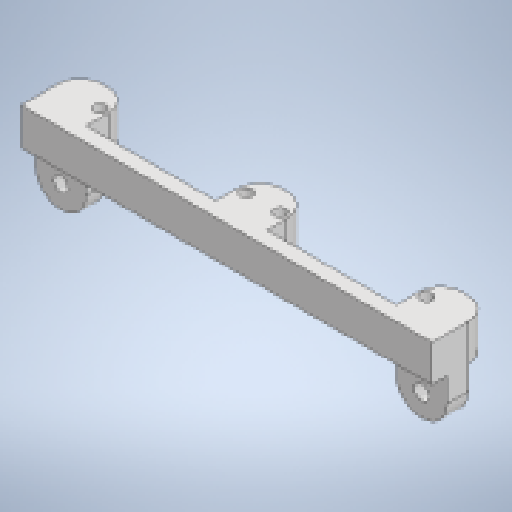
# Autodesk Inventor part: mocowanie_serw
Saved by Autodesk Inventor 2023 (Build 270158000, 158)
## iProperties
Created: 2023-04-06
Part Number: mocowanie_serw
Material: Ogólny
Document SubType Name: Modeling
Designer: Kamil
Density: 1 g/cm^3
Appearance: Domyślna
Author: Kamil
Autodesk Inventor part; units mm, degrees
ref_plane "YZ Plane" through (0, 0, 0) normal (1, 0, 0) x (0, 1, 0)
ref_plane "XZ Plane" through (0, 0, 0) normal (0, 1, 0) x (-1, 0, 0)
ref_plane "XY Plane" through (0, 0, 0) normal (0, 0, 1) x (1, 0, 0)
sketch "Szkic1" plane through (0, 0, 0) normal (0, 0, 1) x (1, 0, 0)
  arc A0 (-14.5572, 8.86) -> (-14.6986, 8.8014) centre (-14.5572, 8.66) ccw projected
  line L0 (-15.5414, 7.9586) -> (-14.6986, 8.8014) projected
  arc A1 (-15.6828, 7.9) -> (-15.5414, 7.9586) centre (-15.6828, 8.1) ccw projected
  line L1 (-16.4, 7.9) -> (-15.6828, 7.9) projected
  line L2 (-16.4, 7.9) -> (-16.4, 6.8) projected
  arc A2 (-16.4, 6.8) -> (-16.2, 6.6) centre (-16.2, 6.8) ccw projected
  line L3 (-16.2, 6.6) -> (-11.8, 6.6) projected
  line L4 (-11.8, 6.6) -> (-11.8, -11.6) projected
  line L5 (-11.8, -11.6) -> (11.8, -11.6) projected
  line L6 (11.8, -11.6) -> (11.8, 6.6) projected
  line L7 (11.8, 6.6) -> (16.2, 6.6) projected
  arc A3 (16.2, 6.6) -> (16.4, 6.8) centre (16.2, 6.8) ccw projected
  line L8 (16.4, 6.8) -> (16.4, 7.9) projected
  line L9 (16.4, 7.9) -> (15.7657, 7.9) projected
  arc A4 (15.4828, 8.0172) -> (15.7657, 7.9) centre (15.7657, 8.3) ccw projected
  line L10 (15.4828, 8.0172) -> (14.6986, 8.8014) projected
  arc A5 (14.6986, 8.8014) -> (14.5572, 8.86) centre (14.5572, 8.66) ccw projected
  line L11 (11.8, 8.86) -> (14.5572, 8.86) projected
  line L12 (11.8, 8.86) -> (11.8, 11.6) projected
  line L13 (11.8, 11.6) -> (8.3794, 11.6) projected
  line L14 (8.3794, 11.6) -> (8.3794, 16) projected
  line L15 (8.3794, 16) -> (4.0206, 16) projected
  line L16 (4.0206, 11.6) -> (4.0206, 16) projected
  line L17 (4.0206, 11.6) -> (-11.8, 11.6) projected
  line L18 (-11.8, 11.6) -> (-11.8, 8.86) projected
  line L19 (-11.8, 8.86) -> (-14.5572, 8.86) projected
  arc A6 (51.4986, 8.8014) -> (51.3572, 8.86) centre (51.3572, 8.66) ccw projected
  line L20 (48.6, 8.86) -> (51.3572, 8.86) projected
  line L21 (48.6, 11.6) -> (48.6, 8.86) projected
  line L22 (32.7794, 11.6) -> (48.6, 11.6) projected
  line L23 (32.7794, 11.6) -> (32.7794, 16) projected
  line L24 (28.4206, 16) -> (32.7794, 16) projected
  line L25 (28.4206, 11.6) -> (28.4206, 16) projected
  line L26 (25, 11.6) -> (28.4206, 11.6) projected
  line L27 (25, 8.86) -> (25, 11.6) projected
  line L28 (25, 8.86) -> (22.2428, 8.86) projected
  arc A7 (22.2428, 8.86) -> (22.1014, 8.8014) centre (22.2428, 8.66) ccw projected
  line L29 (21.3172, 8.0172) -> (22.1014, 8.8014) projected
  arc A8 (21.0343, 7.9) -> (21.3172, 8.0172) centre (21.0343, 8.3) ccw projected
  line L30 (20.4, 7.9) -> (21.0343, 7.9) projected
  line L31 (20.4, 6.8) -> (20.4, 7.9) projected
  arc A9 (20.4, 6.8) -> (20.6, 6.6) centre (20.6, 6.8) ccw projected
  line L32 (25, 6.6) -> (20.6, 6.6) projected
  line L33 (25, -11.6) -> (25, 6.6) projected
  line L34 (48.6, -11.6) -> (25, -11.6) projected
  line L35 (48.6, 6.6) -> (48.6, -11.6) projected
  line L36 (53, 6.6) -> (48.6, 6.6) projected
  arc A10 (53, 6.6) -> (53.2, 6.8) centre (53, 6.8) ccw projected
  line L37 (53.2, 7.9) -> (53.2, 6.8) projected
  line L38 (53.2, 7.9) -> (52.4828, 7.9) projected
  arc A11 (52.3414, 7.9586) -> (52.4828, 7.9) centre (52.4828, 8.1) ccw projected
  line L39 (52.3414, 7.9586) -> (51.4986, 8.8014) projected
  line L40 (-23.6, -41.4743) -> (-23.6, 10.2735) projected
  line L41 (60.4, -41.4743) -> (60.4, 10.2735) projected
  line L42 (-12.3, 19.2958) -> (-12.3, -9.7042) projected
  line L43 (-12.1464, 6.4) -> (-16.2, 6.4) projected
  line L44 (11.8, 6.6) -> (16.2, 6.6) projected
  line L45 (16.2, 6.4) -> (12.1464, 6.4) projected
  line L46 (12.2, 6.4) -> (12.2, -11.6) projected
  line L47 (24.6, 6.4) -> (24.6, -11.6) projected
  line L48 (20.6, 6.4) -> (24.6536, 6.4) projected
  line L49 (12.2, 6.4) -> (24.6, 6.4)
  line L50 (24.6, 6.4) -> (24.6, -11.6)
  line L51 (24.6, -11.6) -> (12.2, -11.6)
  line L52 (12.2, -11.6) -> (12.2, 6.4)
  line L53 (-12.3, 6.4) -> (-23.6, 6.4)
  line L54 (-23.6, 6.4) -> (-23.6, -11.6)
  line L55 (-23.6, -11.6) -> (-12.3, -11.6)
  line L56 (-12.3, -11.6) -> (-12.3, 6.4)
  line L57 (18.4, 10.2735) -> (18.4, 28.3356)
  line L58 (49.1, 6.4) -> (60.4, 6.4)
  line L59 (60.4, 6.4) -> (60.4, -11.6)
  line L60 (60.4, -11.6) -> (49.1, -11.6)
  line L61 (49.1, -11.6) -> (49.1, 6.4)
  line L62 (59.4, 5.4) -> (50.1, 5.4)
  line L63 (50.1, 5.4) -> (50.1, -10.6)
  line L64 (50.1, -10.6) -> (59.4, -10.6)
  line L65 (59.4, -10.6) -> (59.4, 5.4)
  line L66 (13.2, -10.6) -> (23.6, -10.6)
  line L67 (23.6, -10.6) -> (23.6, 5.4)
  line L68 (23.6, 5.4) -> (13.2, 5.4)
  line L69 (13.2, 5.4) -> (13.2, -10.6)
  line L70 (-13.3, -10.6) -> (-22.6, -10.6)
  line L71 (-22.6, -10.6) -> (-22.6, 5.4)
  line L72 (-22.6, 5.4) -> (-13.3, 5.4)
  line L73 (-13.3, 5.4) -> (-13.3, -10.6)
  line L74 (59.4, -10.6) -> (62.4536, -10.6)
  line L75 (59.4, 5.4) -> (62.0484, 5.4)
  line L76 (-22.6, -10.6) -> (-26.8003, -10.6)
  line L77 (-22.6, 5.4) -> (-29.2872, 5.4)
  point P0 (0, 0)
  point P1 (60.4, -10.6)
  point P2 (60.4, 5.4)
  point P3 (-23.6, 5.4)
  point P4 (-23.6, -10.6)
  dimension "d0" = 1
  dimension "d1" = 1
  dimension "d2" = 1
  constraints: 58 end point, 8 parallel, 5 horizontal, 5 perpendicular, 4 symmetric about line, 3 point on line, 1 vertical, 9 other
  measures "d0" distance between parallel lines of L58 L62
  measures "d1" distance between parallel lines of L51 L66
  measures "d2" distance between parallel lines of L55 L70
ref_plane "Płaszczyzna konstrukcyjna1" through (20.4, -11.6, -9) normal (0, 0, -1) x (0, 1, 0)
extrude "Wyciągnięcie proste1" add sketch "Szkic1" against normal up to surface (9 mm away) contours L40 L77 L71 L76 | L71 L72 L73 L70 | L74 L65 L75 L41 | L64 L63 L62 L65 | L69 L68 L67 L66
sketch "Szkic2" plane through (0, 0, 0) normal (0, 0, 1) x (1, 0, 0)
  line L0 (-23.6, 5.4) -> (-23.6, -10.6) projected
  line L1 (-23.6, -10.6) -> (-13.3, -10.6) projected
  line L2 (-13.3, -10.6) -> (-13.3, 5.4) projected
  line L3 (-13.3, 5.4) -> (-23.6, 5.4) projected
  line L4 (50.1, 5.4) -> (50.1, -10.6) projected
  line L5 (50.1, -10.6) -> (60.4, -10.6) projected
  line L6 (60.4, -10.6) -> (60.4, 5.4) projected
  line L7 (60.4, 5.4) -> (50.1, 5.4) projected
  line L8 (23.6, -10.6) -> (23.6, 5.4) projected
  line L9 (23.6, 5.4) -> (13.2, 5.4) projected
  line L10 (13.2, 5.4) -> (13.2, -10.6) projected
  line L11 (13.2, -10.6) -> (23.6, -10.6) projected
  line L12 (-23.6, -10.6) -> (60.4, -10.6)
  line L13 (60.4, -10.6) -> (60.4, 5.4)
  line L14 (60.4, 5.4) -> (-23.6, 5.4)
  line L15 (-23.6, 5.4) -> (-23.6, -10.6)
  point P0 (0, 0)
  constraints: 8 end point, 2 parallel, 1 horizontal, 1 perpendicular
ref_plane "Płaszczyzna konstrukcyjna2" through (60.4, -41.4743, 3) normal (0, 0, 1) x (1, 0, 0)
extrude "Wyciągnięcie proste2" add sketch "Szkic2" along normal up to surface (3 mm away)
sketch "Szkic3" plane through (13.2, -10.6, -9) normal (0, -1, 0) x (1, 0, 0)
  line L0 (36.9, 0) -> (47.2, 0) projected
  line L1 (47.2, 0) -> (47.2, 12) projected
  line L2 (47.2, 12) -> (-36.8, 12) projected
  line L3 (-36.8, 0) -> (-36.8, 12) projected
  line L4 (-36.8, 0) -> (-26.5, 0) projected
  line L5 (-26.5, 9) -> (-26.5, 0) projected
  line L6 (-26.5, 9) -> (0, 9) projected
  line L7 (0, 9) -> (0, 0) projected
  line L8 (0, 0) -> (10.4, 0) projected
  line L9 (10.4, 9) -> (10.4, 0) projected
  line L10 (10.4, 9) -> (36.9, 9) projected
  line L11 (36.9, 9) -> (36.9, 0) projected
  point P0 (-13.2, 9)
extrude "Wyciągnięcie proste3" cut sketch "Szkic3" against normal blind 5
move faces "Przesuń1" translate (0, 1, 0) faces at (28.9667, -5.6, 2)
sketch "Szkic4" plane through (-23.6, -4.6, 3) normal (0, -1, 0) x (1, 0, 0)
  line L0 (74.8605, -3) -> (10.8605, -3) projected
  line L1 (36.8, -12) -> (36.8, -3) projected
  line L2 (47.2, -3) -> (47.2, -12) projected
  line L3 (47.2, -12) -> (36.8, -12) projected
  point P0 (23.6, -3)
ref_plane "Płaszczyzna konstrukcyjna3" through (-11.8, -12, -8.6) normal (0, -1, 0) x (1, 0, 0)
extrude "Wyciągnięcie proste4" add sketch "Szkic4" along normal up to surface (7.4 mm away)
move faces "Przesuń2" translate (0, 2.5, 0) faces at (7.8333, -4.6, 2)
sketch "Szkic5" plane through (13.2, -12, 0) normal (0, 0, 1) x (1, 0, 0)
  line L0 (-36.8, 9.9) -> (47.2, 9.9) projected
  line L1 (0, 9.9) -> (0, 0) projected
  line L2 (0, 0) -> (10.4, 0) projected
  line L3 (10.4, 9.9) -> (10.4, 0) projected
  line L4 (10.4, 0) -> (0, 0) projected
  line L5 (5.2, 0) -> (5.2, 7.1911)
  line L6 (0, 4.95) -> (10.4, 4.95)
  line L7 (10.4, 0) -> (10.4, 17.4) projected
  circle A0 centre (5.2, 4.95) radius 1.5
  point P0 (-13.2, 12)
  dimension "d17" = 3
  constraints: 4 end point, 3 midpoint, 1 centre point, 1 horizontal, 1 point on line, 1 vertical
  measures "d17" diameter of A0
extrude "Wyciągnięcie proste5" cut sketch "Szkic5" against normal through all contours A0 L5 L6 | L6 L5 A0 | A0 L5 L6 | L6 L5 A0
sketch "Szkic6" plane through (-23.6, -2.1, 3) normal (0, -1, 0) x (1, 0, 0)
  line L0 (36.8, -3) -> (47.2, -3) projected
  line L1 (73.7, -3) -> (47.2, -3) projected
  line L2 (73.7, -12) -> (73.7, -3) projected
  line L3 (84, -12) -> (73.7, -12) projected
  line L4 (84, 0) -> (84, -12) projected
  line L5 (0, 0) -> (84, 0) projected
  line L6 (0, -12) -> (0, 0) projected
  line L7 (10.3, -12) -> (0, -12) projected
  line L8 (10.3, -3) -> (10.3, -12) projected
  line L9 (36.8, -3) -> (10.3, -3) projected
  line L10 (0, -3) -> (84, -3)
  line L11 (84, -3) -> (84, -12)
  line L12 (84, -12) -> (0, -12)
  line L13 (0, -12) -> (0, -3)
  line L14 (84, -12) -> (84, 0) projected
  line L15 (0, -3) -> (84, -3)
  line L16 (84, -3) -> (84, -7.5)
  line L17 (84, -7.5) -> (0, -7.5)
  line L18 (0, -7.5) -> (0, -3)
  point P0 (23.6, -3)
  point P1 (73.7, -7.5)
  point P2 (73.7, -3)
  point P3 (0, -7.5)
  point P4 (10.3, -7.5)
  constraints: 16 end point, 4 parallel, 2 horizontal, 2 perpendicular, 2 point on line
extrude "Wyciągnięcie proste6" add sketch "Szkic6" along normal up to surface (9.9 mm away) contours L8 L17 L6 L10 | L10 L4 L17 L2
sketch "Szkic7" plane through (13.2, -12, 0) normal (0, 0, 1) x (1, 0, 0)
  circle A0 centre (5.2, 4.95) radius 1.5 projected
  line L0 (0, 0) -> (10.4, 0) projected
  line L1 (10.4, 9.9) -> (10.4, 0) projected
  line L2 (0, 9.9) -> (10.4, 9.9) projected
  line L3 (0, 9.9) -> (0, 0) projected
  point P0 (-13.2, 12)
extrude "Wyciągnięcie proste7" cut sketch "Szkic7" against normal through all
sketch "Szkic8" plane through (-23.6, -2.1, 0) normal (0, 0, 1) x (1, 0, 0)
  line L0 (0, -9.9) -> (10.3, -9.9) projected
  line L1 (10.3, 0) -> (10.3, -9.9) projected
  line L2 (0, 0) -> (10.3, 0) projected
  line L3 (0, 0) -> (0, -9.9) projected
  line L4 (73.7, -9.9) -> (84, -9.9) projected
  line L5 (84, 0) -> (84, -9.9) projected
  line L6 (73.7, 0) -> (84, 0) projected
  line L7 (73.7, 0) -> (73.7, -9.9) projected
  line L8 (10.3, -9.9) -> (0, -9.9) projected
  line L9 (5.15, -9.9) -> (5.15, -8.4)
  line L10 (5.15, -8.4) -> (5.15, -5.4)
  line L11 (84, -9.9) -> (73.7, -9.9) projected
  line L12 (78.85, -9.9) -> (78.85, -5.4)
  circle A0 centre (5.15, -5.4) radius 1.5
  circle A1 centre (78.85, -5.4) radius 1.5
  point P0 (23.6, 2.1)
  dimension "d24" = 1.5
  dimension "d25" = 3
  dimension "d26" = 4.5
  dimension "d27" = 3
  dimension "d28" = 3
  constraints: 6 end point, 2 centre point, 2 coincident, 2 midpoint, 2 vertical, 1 point on line
  measures "d24" distance of L9.start L9.end
  measures "d25" distance of L9.end L10.end
  measures "d26" distance of L12.start L12.end
  measures "d27" diameter of A0
  measures "d28" diameter of A1
extrude "Wyciągnięcie proste8" cut sketch "Szkic8" against normal through all contours A0 | A1
fillet "Zaokrąglenie1" radius 5 4 edges at (-23.6, -12, -2.25) (-13.3, -12, -2.25) (50.1, -12, -2.25) (60.4, -12, -2.25)
fillet "Zaokrąglenie2" radius 5 2 edges at (13.2, 1.65, -9) (23.6, 1.65, -9)
fillet "Zaokrąglenie3" radius 4.5 4 edges at (-23.6, 1.65, -9) (-13.3, 1.65, -9) (50.1, 1.65, -9) (60.4, 1.65, -9)
sketch "Szkic9" plane through (23.6, 5.4, 0) normal (0, 1, 0) x (1, 0, 0)
  arc A0 (36.8, 4.5) -> (32.3, 9) centre (32.3, 4.5) ccw projected
  line L0 (32.3, 9) -> (31, 9) projected
  arc A1 (31, 9) -> (26.5, 4.5) centre (31, 4.5) ccw projected
  line L1 (26.5, 0) -> (26.5, 4.5) projected
  line L2 (26.5, 0) -> (0, 0) projected
  line L3 (0, 0) -> (0, 4) projected
  arc A2 (0, 4) -> (-5, 9) centre (-5, 4) ccw projected
  line L4 (-5, 9) -> (-5.4, 9) projected
  arc A3 (-5.4, 9) -> (-10.4, 4) centre (-5.4, 4) ccw projected
  line L5 (-10.4, 0) -> (-10.4, 4) projected
  line L6 (-10.4, 0) -> (-36.9, 0) projected
  line L7 (-36.9, 0) -> (-36.9, 4.5) projected
  arc A4 (-36.9, 4.5) -> (-41.4, 9) centre (-41.4, 4.5) ccw projected
  line L8 (-41.4, 9) -> (-42.7, 9) projected
  arc A5 (-42.7, 9) -> (-47.2, 4.5) centre (-42.7, 4.5) ccw projected
  line L9 (-47.2, -3) -> (-47.2, 4.5) projected
  line L10 (-47.2, -3) -> (36.8, -3) projected
  line L11 (36.8, 4.5) -> (36.8, -3) projected
  line L12 (28.8828, 7.5) -> (28.8828, 9) projected
  line L13 (25.4, 7.5) -> (28.8828, 7.5) projected
  line L14 (25.4, 1.5) -> (25.4, 7.5) projected
  line L15 (25.4, 1.5) -> (28.8828, 1.5) projected
  line L16 (28.8828, 0) -> (28.8828, 1.5) projected
  line L17 (29.6, 0) -> (28.8828, 0) projected
  line L18 (29.6, 2.75) -> (29.6, 0) projected
  line L19 (29.6, 2.75) -> (28.15, 2.75) projected
  arc A6 (28.15, 6.25) -> (28.15, 2.75) centre (28.15, 4.5) ccw projected
  line L20 (28.15, 6.25) -> (29.6, 6.25) projected
  line L21 (29.6, 9) -> (29.6, 6.25) projected
  line L22 (28.8828, 9) -> (29.6, 9) projected
  line L23 (-3.2, 0) -> (-3.2, 2.75) projected
  line L24 (-3.2, 0) -> (-2.5657, 0) projected
  line L25 (-2.5657, 1.5) -> (-2.5657, 0) projected
  line L26 (1, 1.5) -> (-2.5657, 1.5) projected
  line L27 (1, 7.5) -> (1, 1.5) projected
  line L28 (1, 7.5) -> (-2.5657, 7.5) projected
  line L29 (-2.5657, 9) -> (-2.5657, 7.5) projected
  line L30 (-2.5657, 9) -> (-3.2, 9) projected
  line L31 (-3.2, 6.25) -> (-3.2, 9) projected
  line L32 (-1.75, 6.25) -> (-3.2, 6.25) projected
  arc A7 (-1.75, 2.75) -> (-1.75, 6.25) centre (-1.75, 4.5) ccw projected
  line L33 (-3.2, 2.75) -> (-1.75, 2.75) projected
  line L34 (-7.2, 0) -> (-7.2, 2.75) projected
  line L35 (-7.2, 2.75) -> (-8.65, 2.75) projected
  arc A8 (-8.65, 6.25) -> (-8.65, 2.75) centre (-8.65, 4.5) ccw projected
  line L36 (-8.65, 6.25) -> (-7.2, 6.25) projected
  line L37 (-7.2, 6.25) -> (-7.2, 9) projected
  line L38 (-7.8343, 9) -> (-7.2, 9) projected
  line L39 (-7.8343, 9) -> (-7.8343, 7.5) projected
  line L40 (-11.4, 7.5) -> (-7.8343, 7.5) projected
  line L41 (-11.4, 7.5) -> (-11.4, 1.5) projected
  line L42 (-11.4, 1.5) -> (-7.8343, 1.5) projected
  line L43 (-7.8343, 1.5) -> (-7.8343, 0) projected
  line L44 (-7.2, 0) -> (-7.8343, 0) projected
  line L45 (-39.2828, 7.5) -> (-39.2828, 9) projected
  line L46 (-39.2828, 9) -> (-40, 9) projected
  line L47 (-40, 9) -> (-40, 6.25) projected
  line L48 (-38.55, 6.25) -> (-40, 6.25) projected
  arc A9 (-38.55, 2.75) -> (-38.55, 6.25) centre (-38.55, 4.5) ccw projected
  line L49 (-40, 2.75) -> (-38.55, 2.75) projected
  line L50 (-40, 2.75) -> (-40, 0) projected
  line L51 (-40, 0) -> (-39.2828, 0) projected
  line L52 (-39.2828, 0) -> (-39.2828, 1.5) projected
  line L53 (-35.8, 1.5) -> (-39.2828, 1.5) projected
  line L54 (-35.8, 1.5) -> (-35.8, 7.5) projected
  line L55 (-35.8, 7.5) -> (-39.2828, 7.5) projected
  circle A10 centre (-8.65, 4.5) radius 1.25
  circle A11 centre (-1.75, 4.5) radius 1.25
  circle A12 centre (-38.55, 4.5) radius 1.25
  circle A13 centre (28.15, 4.5) radius 1.25
  point P0 (-23.6, 0)
  dimension "d34" = 2.5
  dimension "d35" = 2.5
  dimension "d36" = 2.5
  dimension "d37" = 2.5
  constraints: 4 centre point, 4 coincident
  measures "d34" diameter of A10
  measures "d35" diameter of A11
  measures "d36" diameter of A12
  measures "d37" diameter of A13
extrude "Wyciągnięcie proste9" cut sketch "Szkic9" against normal through all contours A10 | A11 | A12 | A13
sketch "Szkic10" plane through (-23.6, -2.1, 3) normal (-1, 0, 0) x (0, 0, 1)
  circle A0 centre (-3.75, 3.75) radius 1.7 projected
  point P0 (-3, 2.1)
extrude "Wyciągnięcie proste10" cut sketch "Szkic10" against normal blind 8
